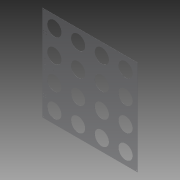
# Autodesk Inventor part: Plastic Funnel PIece
Saved by Autodesk Inventor 2014 (Build 180170000, 170)
## iProperties
Created: 2014-01-04
Part Number: Plastic Funnel PIece
Material: Polycarbonate, Clear
Document SubType Name: Sheet Metal
Designer: Michael
Density: 1.2 g/cm^3
Appearance: Polycarbonate - Clear
Sheet Metal Rule: Default
Mass: 176.028 g
Surface Area: 3744.52 cm^2
Volume: 146.69 cm^3
Author: Michael
Autodesk Inventor part; units mm, degrees
ref_plane "YZ Plane" through (0, 0, 0) normal (1, 0, 0) x (0, 1, 0)
ref_plane "XZ Plane" through (0, 0, 0) normal (0, 1, 0) x (-1, 0, 0)
ref_plane "XY Plane" through (0, 0, 0) normal (0, 0, 1) x (1, 0, 0)
sketch "Sketch1" plane through (0, 0, 0) normal (0, 0, 1) x (1, 0, 0)
  line L0 (0, 0) -> (508, 0)
  line L1 (508, 0) -> (508, 508)
  line L2 (508, 508) -> (0, 508)
  line L3 (0, 508) -> (0, 0)
  line L4 (0, 254) -> (508, 254) construction
  line L5 (254, 508) -> (254, 0) construction
  line L6 (25.4, 482.6) -> (482.6, 482.6) construction
  line L7 (482.6, 482.6) -> (482.6, 25.4) construction
  line L8 (482.6, 25.4) -> (25.4, 25.4) construction
  line L9 (25.4, 25.4) -> (25.4, 482.6) construction
  circle A0 centre (6.35, 501.65) radius 2.4892
  circle A1 centre (501.65, 501.65) radius 2.4892
  circle A2 centre (501.65, 6.35) radius 2.4892
  circle A3 centre (6.35, 6.35) radius 2.4892
  line L10 (254, 254) -> (25.4, 254) construction
  circle A4 centre (6.35, 406.4) radius 2.4892
  circle A5 centre (6.35, 393.7) radius 2.4892
  circle A6 centre (19.05, 406.4) radius 2.4892
  circle A7 centre (19.05, 393.7) radius 2.4892
  circle A8 centre (6.35, 101.6) radius 2.4892
  circle A9 centre (6.35, 114.3) radius 2.4892
  circle A10 centre (19.05, 101.6) radius 2.4892
  circle A11 centre (19.05, 114.3) radius 2.4892
  line L11 (0, 292.1) -> (19.05, 292.1) construction
  line L12 (19.05, 292.1) -> (19.05, 215.9) construction
  line L13 (19.05, 215.9) -> (0, 215.9) construction
  line L14 (0, 215.9) -> (0, 292.1) construction
  circle A12 centre (12.7, 279.4) radius 2.4892
  circle A13 centre (12.7, 228.6) radius 2.4892
  circle A14 centre (12.7, 254) radius 2.4892
  dimension "d5" = 508
  dimension "d6" = 508
  dimension "d12" = 25.4
  dimension "d67" = 4.9784
  dimension "d69" = 6.35
  dimension "d70" = 6.35
  dimension "d106" = 4.9784
  dimension "d109" = 12.7
  dimension "d112" = 12.7
  dimension "d115" = 6.35
  dimension "d116" = 101.6
  dimension "d117" = 19.05
  dimension "d118" = 76.2
  dimension "d119" = 4.9784
  dimension "d120" = 12.7
  dimension "d121" = 6.35
  dimension "d123" = 6.35
  constraints: 30 end point, 15 centre point, 8 symmetric about line, 6 midpoint, 6 parallel, 3 horizontal, 3 perpendicular, 2 point on line, 1 equal radius, 1 vertical, 18 other
  measures "d5" distance of L2.end L1.end
  measures "d6" distance of L1.end L0.end
  measures "d12" distance between parallel lines of L6 L2
  measures "d67" diameter of A0
  measures "d69" distance from line of L2 A0.centre
  measures "d70" distance from line of L3 A0.centre
  measures "d106" diameter of A4
  measures "d109" distance of A4.centre A5.centre
  measures "d112" distance of A4.centre A6.centre
  measures "d115" distance from line of L3 A4.centre
  measures "d116" distance from line of L2 A4.centre
  measures "d117" distance of L12.end L13.end
  measures "d118" distance of L11.end L12.end
  measures "d119" diameter of A12
  measures "d120" distance from line of L11 A12.centre
  measures "d121" distance from line of L12 A12.centre
  measures "d123" distance from line of L12 A14.centre
extrude "Extrusion1" add sketch "Sketch1" along normal blind 0.7937
sketch "Sketch3" plane through (0, 0, 0) normal (0, 0, -1) x (-1, 0, 0)
  line L0 (-508, 508) -> (0, 508) projected
  line L1 (-508, 0) -> (-508, 508) projected
  circle A0 centre (-444.5, 444.5) radius 38.1
  dimension "d26" = 76.2
  dimension "d27" = 63.5
  dimension "d28" = 63.5
  constraints: 1 centre point
  measures "d26" diameter of A0
  measures "d27" distance from line of L0 A0.centre
  measures "d28" distance from line of L1 A0.centre
extrude "Extrusion3" cut sketch "Sketch3" against normal blind 1.5875
pattern_linear "Rectangular Pattern1" count 4 spacing 127 along (-1, 0, 0) count 4 spacing 127 along (0, -1, 0) of "Extrusion3"
sketch "Sketch4" plane through (0, 0, 0.7937) normal (0, 0, 1) x (1, 0, 0)
  circle A0 centre (12.7, 254) radius 2.4892 projected
  line L0 (508, 0) -> (508, 508) projected
  line L1 (0, 508) -> (0, 0) projected
  line L2 (63.5, 266.7) -> (50.8, 266.7) construction
  line L3 (50.8, 266.7) -> (50.8, 241.3) construction
  line L4 (50.8, 241.3) -> (63.5, 241.3) construction
  line L5 (63.5, 241.3) -> (63.5, 266.7) construction
  line L6 (0, 254) -> (508, 254) construction
  circle A1 centre (57.15, 260.35) radius 2.4892
  circle A2 centre (57.15, 247.65) radius 2.4892
  dimension "d124" = 25.4
  dimension "d125" = 12.7
  dimension "d126" = 4.9784
  dimension "d127" = 6.35
  dimension "d130" = 50.8
  dimension "d131" = 6.35
  constraints: 10 end point, 2 centre point, 2 midpoint, 2 parallel, 2 perpendicular, 1 horizontal, 1 point on line, 1 symmetric about line, 2 other
  measures "d124" distance of L2.end L3.end
  measures "d125" distance of L3.end L4.end
  measures "d126" diameter of A1
  measures "d127" distance from line of L2 A1.centre
  measures "d130" distance between parallel lines of L1 L3
  measures "d131" distance from line of A1.centre L3
extrude "Extrusion4" cut sketch "Sketch4" against normal blind 25.4 contours A1 | A2
equation "\"BendRadius\" = Thickness"
equation "\"BendReliefWidth\" = Thickness"
equation "\"BendReliefDepth\" = 0.5 * Thickness"
equation "\"CornerReliefSize\" = 4 * Thickness"
equation "\"MinimumRemnant\" = 2 * Thickness"
equation "\"TransitionRadius\" = BendRadius"
equation "\"JacobiRadiusSize\" = Thickness"
equation "\"GapSize\" = Thickness"
equation "\"Thickness\" = 3.048"
body "Solid2"
